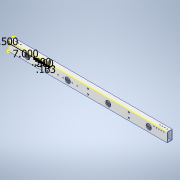
# Autodesk Inventor part: Chassis side 1
Saved by Autodesk Inventor 2022 (Build 260153000, 153)
## iProperties
Created: 2022-11-14
Part Number: Chassis side 1
Material: Aluminum 6061
Document SubType Name: Modeling
Designer: s135320
Density: 2.7 g/cm^3
Appearance: Aluminum - Flat
Mass: 869.998 g
Surface Area: 2079.03 cm^2
Volume: 322.222 cm^3
Author: s135320
Autodesk Inventor part; units mm, degrees
ref_plane "YZ Plane" through (0, 0, 0) normal (1, 0, 0) x (0, 1, 0)
ref_plane "XZ Plane" through (0, 0, 0) normal (0, 1, 0) x (-1, 0, 0)
ref_plane "XY Plane" through (0, 0, 0) normal (0, 0, 1) x (1, 0, 0)
sketch "Sketch1" plane through (0, 0, 0) normal (0, 1, 0) x (-1, 0, 0)
  point P0 (0, 0)
sketch "Sketch2" plane through (0, 0, 0) normal (0, 0, 1) x (1, 0, 0)
  line L0 (0, 0) -> (838.2, 0)
  line L1 (838.2, 0) -> (838.2, 50.8)
  line L2 (838.2, 50.8) -> (0, 50.8)
  line L3 (0, 50.8) -> (0, 0)
  circle A0 centre (740.5688, 25.4) radius 14.2875
  circle A1 centre (97.6371, 25.4) radius 14.2875
  line L4 (0, 25.4) -> (838.2, 25.4) construction
  circle A2 centre (311.9438, 23.8125) radius 14.2875
  circle A3 centre (288.1313, 23.8125) radius 2.159
  circle A4 centre (335.7563, 23.8125) radius 2.159
  circle A5 centre (362.7438, 23.8125) radius 2.54
  circle A6 centre (261.1438, 23.8125) radius 2.54
  circle A7 centre (327.8188, 23.8125) radius 7.9375 construction
  line L5 (97.6371, 25.4) -> (97.6371, 90.8259)
  line L6 (740.5688, 25.4) -> (740.5688, 86.7676)
  line L7 (327.8188, 23.8125) -> (327.8188, 91.6838)
  circle A8 centre (526.2563, 23.8125) radius 14.2875
  line L8 (526.2563, 23.8125) -> (327.8188, 23.8125)
  line L9 (97.6371, 25.4) -> (97.6371, 0) construction
  line L10 (311.9438, 23.8125) -> (311.9438, 0) construction
  line L11 (526.2563, 23.8125) -> (526.2563, 0) construction
  line L12 (740.5688, 25.4) -> (740.5687, 0) construction
  line L13 (740.5687, 0) -> (526.2563, 0) construction
  line L14 (311.9438, 0) -> (355.3784, 0)
  line L15 (526.2563, 0) -> (311.9438, 0) construction
  line L16 (97.6371, 0) -> (311.9438, 0) construction
  line L17 (204.7904, 0) -> (204.7904, 50.8) construction
  line L18 (633.4125, 0) -> (633.4125, 50.8) construction
  line L19 (419.1, 0) -> (419.1, 50.8) construction
  line L20 (526.2563, 0) -> (419.1, 0) construction
  line L21 (0, 25.4) -> (0, 0) construction
  line L22 (0, 25.4) -> (0, 50.8) construction
  line L23 (0, 38.1) -> (838.2, 38.1) construction
  line L24 (0, 0) -> (0, 25.4) construction
  line L25 (0, 12.7) -> (838.2, 12.7) construction
  circle A9 centre (419.1, 38.1) radius 3.81
  circle A10 centre (419.1, 12.7) radius 3.81
  line L26 (311.9438, 23.8125) -> (526.2563, 23.8125)
  line L27 (419.1, 23.8125) -> (419.1, 31.9987)
  circle A11 centre (203.2, 38.1) radius 3.81
  circle A12 centre (203.2, 12.7) radius 3.81
  circle A13 centre (635, 38.1) radius 3.81
  circle A14 centre (635, 12.7) radius 3.81
  point P0 (190.5066, 50.8)
  dimension "d0" = 50.8
  dimension "d1" = 838.2
  dimension "d9" = 28.575
  dimension "d10" = 28.575
  dimension "d13" = 23.8125
  dimension "d14" = 23.8125
  dimension "d17" = 28.575
  dimension "d18" = 4.318
  dimension "d19" = 4.318
  dimension "d20" = 50.8
  dimension "d21" = 50.8
  dimension "d22" = 5.08
  dimension "d23" = 5.08
  dimension "d70" = 214.3125
  dimension "d72" = 28.575
  dimension "d73" = 214.3125
  dimension "d74" = 214.3125
  dimension "d99" = 7.62
  dimension "d100" = 7.62
  dimension "d113" = 419.1
  dimension "d114" = 1.5875
  dimension "d116" = 7.62
  dimension "d117" = 7.62
  dimension "d118" = 7.62
  dimension "d119" = 7.62
  dimension "d120" = 203.2
  dimension "d121" = 203.2
  dimension "d122" = 203.2
  dimension "d123" = 203.2
  constraints: 56 end point, 19 point on line, 14 centre point, 12 perpendicular, 11 midpoint, 6 collinear, 4 parallel, 1 horizontal, 1 horizontal alignment, 2 other
  measures "d0" distance of L2.end L0.start
  measures "d1" distance of L1.end L2.end
  measures "d9" diameter of A0
  measures "d10" diameter of A1
  measures "d13" distance of A4.centre L10.start
  measures "d14" distance of L10.start A3.centre
  measures "d17" diameter of A2
  measures "d18" diameter of A3
  measures "d19" diameter of A4
  measures "d20" distance of L10.start A6.centre
  measures "d21" distance of A5.centre L10.start
  measures "d22" diameter of A6
  measures "d23" diameter of A5
  measures "d70" distance of L5.start L10.start
  measures "d72" diameter of A8
  measures "d73" distance of L10.start L8.start
  measures "d74" horizontal distance of L8.start L6.start
  measures "d99" diameter of A9
  measures "d100" diameter of A10
  measures "d113" distance from line of L3 L27.start
  measures "d114" distance from line of L4 L10.start
  measures "d116" diameter of A12
  measures "d117" diameter of A11
  measures "d118" diameter of A13
  measures "d119" diameter of A14
  measures "d120" distance from line of L1 A13.centre
  measures "d121" distance from line of L1 A14.centre
  measures "d122" distance from line of A11.centre L3
  measures "d123" distance from line of A12.centre L3
extrude "Extrusion1" add sketch "Sketch2" along normal blind 25.4 contours L3 L2 L1 L0 | A0 | A1 | A2 | A3 | L8 A4 | A4 L8 | L8 A5 | A5 L8 | A6 | A8 | A9 | A10 | A11 | A12 | A13 | A14
shell "Shell1" thickness 3.175 removed faces 2 at (838.2, 16.9333, 8.4667) at (0, 33.8667, 16.9333)
extrude "Extrusion2" cut sketch "Sketch2" along normal blind 174.9425 contours A0 | A1 | A2 | A3 | L8 A4 | A4 L8 | L8 A5 | A5 L8 | A6 | A8 | A9 | A10 | A11 | A12 | A13 | A14
sketch "Sketch3" plane through (0, 0, 0) normal (0, 0, -1) x (-1, 0, 0)
  circle A0 centre (-261.1438, 23.8125) radius 2.54 projected
  circle A1 centre (-362.7438, 23.8125) radius 2.54 projected
  circle A2 centre (-362.7438, 23.8125) radius 2.54 projected
  circle A3 centre (-362.7438, 23.8125) radius 4.445
  circle A4 centre (-261.1438, 23.8125) radius 4.445
  point P0 (0, 0)
  dimension "d29" = 8.89
  dimension "d30" = 8.89
  constraints: 2 centre point, 2 coincident
  measures "d29" diameter of A4
  measures "d30" diameter of A3
extrude "Extrusion3" cut sketch "Sketch3" against normal up to surface (22.225 mm away) contours A0 | A3 | A4
sketch "Sketch5" plane through (0, 50.8, 0) normal (0, 1, 0) x (1, 0, 0)
  point P0 (0, 0)
sketch "Sketch6" plane through (0, 50.8, 0) normal (0, 1, 0) x (1, 0, 0)
  point P0 (0, 0)
sketch "Sketch7" plane through (0, 50.8, 0) normal (0, 1, 0) x (1, 0, 0)
  line L0 (0, -22.225) -> (0, -3.175) construction
  line L1 (0, -12.7) -> (838.2, -12.7) construction
  line L2 (838.2, 0) -> (838.2, -25.4) construction
  circle A0 centre (0, -12.7) radius 2.0701
  circle A1 centre (12.7, -12.7) radius 2.0701
  circle A2 centre (25.4, -12.7) radius 2.0701
  circle A3 centre (38.1, -12.7) radius 2.0701
  circle A4 centre (50.8, -12.7) radius 2.0701
  line L3 (419.1, -12.7) -> (419.1, -25.4) construction
  circle A5 centre (419.1, -12.7) radius 2.0701
  circle A6 centre (431.8, -12.7) radius 2.0701
  circle A7 centre (444.5, -12.7) radius 2.0701
  circle A8 centre (457.2, -12.7) radius 2.0701
  circle A9 centre (406.4, -12.7) radius 2.0701
  circle A10 centre (419.1, -12.7) radius 2.0701
  circle A11 centre (431.8, -12.7) radius 2.0701
  circle A12 centre (444.5, -12.7) radius 2.0701
  circle A13 centre (393.7, -12.7) radius 2.0701
  circle A14 centre (406.4, -12.7) radius 2.0701
  circle A15 centre (419.1, -12.7) radius 2.0701
  circle A16 centre (431.8, -12.7) radius 2.0701
  circle A17 centre (381, -12.7) radius 2.0701
  circle A18 centre (393.7, -12.7) radius 2.0701
  circle A19 centre (406.4, -12.7) radius 2.0701
  circle A20 centre (419.1, -12.7) radius 2.0701
  circle A21 centre (825.5, -12.7) radius 2.0701
  circle A22 centre (812.8, -12.7) radius 2.0701
  circle A23 centre (800.1, -12.7) radius 2.0701
  circle A24 centre (787.4, -12.7) radius 2.0701
  point P0 (0, 0)
  dimension "d77" = 4.1402
  dimension "d80" = 12.7
  dimension "d85" = 4.1402
  dimension "d88" = 12.7
  dimension "d91" = 12.7
  constraints: 25 centre point, 4 end point, 4 symmetric about line, 3 horizontal, 3 midpoint, 2 coincident, 1 vertical, 42 other
  measures "d77" diameter of A0
  measures "d80" distance of A0.centre A1.centre
  measures "d85" diameter of A5
  measures "d88" distance of A5.centre A6.centre
  measures "d91" distance of A5.centre A9.centre
extrude "Extrusion5" cut sketch "Sketch7" against normal through all contours A1 | A2 | A3 | A4 | A21 | A22 | A23 | A24
sketch "Sketch8" plane through (0, 0, 25.4) normal (0, 0, 1) x (1, 0, 0)
  point P0 (0, 0)
sketch "Sketch9" plane through (0, 0, 25.4) normal (0, 0, 1) x (1, 0, 0)
  line L0 (0, 0) -> (838.2, 0) projected
  line L1 (838.2, 0) -> (819.15, 0)
  line L2 (819.15, 0) -> (819.15, 50.8)
  line L3 (838.2, 50.8) -> (0, 50.8) projected
  line L4 (819.15, 50.8) -> (819.15, 53.2892)
  line L5 (819.15, 53.2892) -> (819.15, 41.2718)
  line L6 (819.15, 53.2892) -> (819.15, 40.5892)
  line L7 (819.15, 40.5892) -> (806.45, 40.5892)
  circle A0 centre (819.15, 40.5892) radius 2.0701
  circle A1 centre (806.45, 40.5892) radius 2.0701
  circle A2 centre (793.75, 40.5892) radius 2.0701
  circle A3 centre (781.05, 40.5892) radius 2.0701
  circle A4 centre (768.35, 40.5892) radius 2.0701
  dimension "d124" = 19.05
  dimension "d125" = 2.4892
  dimension "d126" = 12.7
  dimension "d127" = 12.7
  dimension "d128" = 4.1402
  dimension "d131" = 12.7
  constraints: 12 end point, 5 centre point, 5 point on line, 1 coincident, 1 horizontal, 1 perpendicular, 1 vertical, 8 other
  measures "d124" distance of L0.end L1.end
  measures "d125" distance of L2.end L4.end
  measures "d126" distance of L4.end L6.end
  measures "d127" distance of L6.end L7.end
  measures "d128" diameter of A0
  measures "d131" distance of A0.centre A1.centre
extrude "Extrusion6" cut sketch "Sketch9" against normal through all
sketch "Sketch10" plane through (0, 0, 25.4) normal (0, 0, 1) x (1, 0, 0)
  line L0 (838.2, 50.8) -> (0, 50.8) projected
  line L1 (0, 50.8) -> (0, 38.1)
  line L2 (0, 47.625) -> (0, 3.175) projected
  line L3 (0, 38.1) -> (177.8, 38.1)
  circle A0 centre (177.8, 38.1) radius 2.0701
  circle A1 centre (190.5, 38.1) radius 2.0701
  circle A2 centre (203.2, 38.1) radius 2.0701
  circle A3 centre (215.9, 38.1) radius 2.0701
  circle A4 centre (165.1, 38.1) radius 2.0701
  circle A5 centre (177.8, 38.1) radius 2.0701
  circle A6 centre (190.5, 38.1) radius 2.0701
  circle A7 centre (203.2, 38.1) radius 2.0701
  circle A8 centre (152.4, 38.1) radius 2.0701
  circle A9 centre (165.1, 38.1) radius 2.0701
  circle A10 centre (177.8, 38.1) radius 2.0701
  circle A11 centre (190.5, 38.1) radius 2.0701
  circle A12 centre (139.7, 38.1) radius 2.0701
  circle A13 centre (152.4, 38.1) radius 2.0701
  circle A14 centre (165.1, 38.1) radius 2.0701
  circle A15 centre (177.8, 38.1) radius 2.0701
  point P0 (0, 0)
  dimension "d138" = 12.7
  dimension "d139" = 177.8
  dimension "d140" = 4.1402
  dimension "d143" = 12.7
  dimension "d146" = 12.7
  constraints: 16 centre point, 4 end point, 2 horizontal, 1 coincident, 1 perpendicular, 1 point on line, 30 other
  measures "d138" distance of L0.end L1.end
  measures "d139" distance of L1.end L3.end
  measures "d140" diameter of A0
  measures "d143" distance of A0.centre A1.centre
  measures "d146" distance of A0.centre A4.centre
equation "\"d70\" = d73"
body "Solid1"
